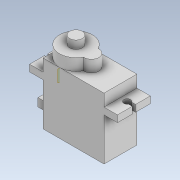
# Autodesk Inventor part: sg90
Saved by Autodesk Inventor 2022.5 (Build 265521000, 521)
## iProperties
Created: 2024-03-15
Part Number: sg90
Material: 常规
Document SubType Name: Modeling
Designer: Gagouking
Density: 1 g/cm^3
Appearance: 默认
Author: Gagouking
Autodesk Inventor part; units mm, degrees
ref_plane "YZ Plane" through (0, 0, 0) normal (1, 0, 0) x (0, 1, 0)
ref_plane "XZ Plane" through (0, 0, 0) normal (0, 1, 0) x (-1, 0, 0)
sketch "草图1" plane through (0, 0, 0) normal (0, 1, 0) x (-1, 0, 0)
  line L0 (0, 0) -> (-22.6, 0)
  line L1 (-22.6, 0) -> (-22.6, 12.2)
  line L2 (-22.6, 12.2) -> (0, 12.2)
  line L3 (0, 12.2) -> (0, 0)
  dimension "d0" = 22.6
  dimension "d1" = 12.2
  constraints: 8 end point, 2 parallel, 1 horizontal, 1 perpendicular
  measures "d0" distance of L1.end L2.end
  measures "d1" distance of L0.end L1.end
extrude "拉伸1" add sketch "草图1" along normal blind 22.8
ref_plane "工作平面1" through (0, 15.8, 0) normal (0, 1, 0) x (1, 0, 0)
sketch "草图2" plane through (0, 15.8, 0) normal (0, 1, 0) x (1, 0, 0)
  line L0 (-5, -12.2) -> (27.6, -12.2)
  line L1 (27.6, -12.2) -> (27.6, 0)
  line L2 (27.6, 0) -> (-5, 0)
  line L3 (-5, 0) -> (-5, -12.2)
  line L4 (0, -12.2) -> (22.6, -12.2) projected
  line L5 (22.6, -12.2) -> (22.6, 0) projected
  line L6 (22.6, 0) -> (0, 0) projected
  line L7 (0, 0) -> (0, -12.2) projected
  line L8 (22.6, 0) -> (0, 0) projected
  line L9 (0, -12.2) -> (22.6, -12.2) projected
  dimension "d5" = 5
  dimension "d6" = 5
  constraints: 8 end point, 2 collinear, 2 parallel, 1 horizontal, 1 perpendicular
  measures "d5" distance between parallel lines of L7 L3
  measures "d6" distance between parallel lines of L5 L1
extrude "拉伸2" add sketch "草图2" along normal blind 2.5
sketch "草图3" plane through (0, 22.8, 0) normal (0, 1, 0) x (1, 0, 0)
  line L0 (0, -12.2) -> (22.6, -12.2) projected
  line L1 (22.6, -12.2) -> (22.6, 0) projected
  line L2 (22.6, 0) -> (0, 0) projected
  line L3 (0, 0) -> (0, -12.2) projected
  circle A0 centre (6.1, -6.1) radius 6.1
  line L4 (0, 0) -> (0, -12.2) projected
  line L5 (0, -6.1) -> (6.1, -6.1) construction
  circle A1 centre (11.85, -6.1) radius 2.75
  line L6 (14.6, -6.1) -> (0, -6.1) construction
  point P0 (11.553, -3.3661)
  point P1 (11.553, -8.8339)
  dimension "d14" = 5.5
  dimension "d15" = 14.6
  constraints: 4 end point, 2 horizontal, 2 midpoint, 2 tangent, 1 centre point, 1 coincident, 1 point on line, 3 other
  measures "d15" distance of L6.start L6.end
extrude "拉伸3" add sketch "草图3" along normal blind 4.4 contours A0 A1 | A1 A0 | A0 A1
sketch "草图4" plane through (6.1, 27.2, 6.1) normal (0, 1, 0) x (0, 0, 1)
  arc A0 (-2.7339, 5.453) -> (2.7339, 5.453) centre (0, 0) ccw projected
  circle A1 centre (0, 0) radius 2.35
  arc A2 (2.7339, 5.453) -> (-2.7339, 5.453) centre (0, 5.75) ccw projected
  point P0 (-6.1, -6.1)
  dimension "d16" = 4.7
  constraints: 1 centre point, 1 coincident
  measures "d16" diameter of A1
extrude "拉伸4" add sketch "草图4" along normal blind 3 contours A1
sketch "草图5" plane through (0, 18.3, 0) normal (0, 1, 0) x (1, 0, 0)
  line L0 (0, 0) -> (0, -12.2) projected
  line L1 (0, 0) -> (-5, 0) projected
  line L2 (-5, 0) -> (-5, -12.2) projected
  line L3 (-5, -12.2) -> (0, -12.2) projected
  line L4 (22.6, -12.2) -> (22.6, 0) projected
  line L5 (22.6, -12.2) -> (27.6, -12.2) projected
  line L6 (27.6, -12.2) -> (27.6, 0) projected
  line L7 (27.6, 0) -> (22.6, 0) projected
  circle A0 centre (-2.5, -6.1) radius 1.25
  circle A1 centre (25.1, -6.1) radius 1.25
  line L8 (-5, 0) -> (-5, -12.2) projected
  line L9 (-5, -6.1) -> (-2.5, -6.1) construction
  line L10 (-5, -6.7) -> (-3.5966, -6.7)
  line L11 (-5, -5.5) -> (-3.5966, -5.5)
  line L12 (27.6, -12.2) -> (27.6, 0) projected
  line L13 (27.6, -6.7) -> (26.1966, -6.7)
  line L14 (27.6, -5.5) -> (26.1966, -5.5)
  point P0 (0, 0)
  dimension "d17" = 2.5
  dimension "d18" = 2.5
  dimension "d19" = 2.5
  dimension "d20" = 2.5
  dimension "d21" = 0.6
  dimension "d22" = 0.6
  constraints: 10 end point, 4 symmetric about line, 3 horizontal, 3 point on line, 1 coincident, 1 midpoint, 6 other
  measures "d19" distance from line of L6 point (25.1, -6.1)
  measures "d20" distance from line of L2 point (-2.5, -6.1)
  measures "d21" distance between parallel lines of L9 L10
  measures "d22" distance between parallel lines of L9 L13
extrude "拉伸5" cut sketch "草图5" against normal through all contours L11 A0 L10 L2 | A0 | L13 A1 L14 L6 | A1
sketch "草图6" plane through (0, 0, 0) normal (-1, 0, 0) x (0, 0, 1)
  line L0 (3.1, 6) -> (9.1, 6)
  line L1 (9.1, 6) -> (9.1, 3)
  line L2 (9.1, 3) -> (3.1, 3)
  line L3 (3.1, 3) -> (3.1, 6)
  line L4 (12.2, 15.8) -> (0, 15.8) projected
  line L5 (0, 0) -> (0, 15.8) projected
  line L6 (0, 0) -> (12.2, 0) projected
  line L7 (12.2, 0) -> (12.2, 15.8) projected
  line L8 (6.1, 0) -> (6.1, 6) construction
  dimension "d25" = 6
  dimension "d26" = 3
  dimension "d27" = 6
  constraints: 10 end point, 2 midpoint, 2 parallel, 1 horizontal, 1 perpendicular, 1 vertical
  measures "d25" distance between parallel lines of L6 L0
  measures "d26" distance of L0.end L1.end
  measures "d27" distance of L1.end L2.end
extrude "拉伸6" add sketch "草图6" along normal blind 5 contours L0 L1 L2 L3
ref_plane "工作平面2" through (6.1, 18.3, 12.2) normal (-1, 0, 0) x (0, 0, 1)
